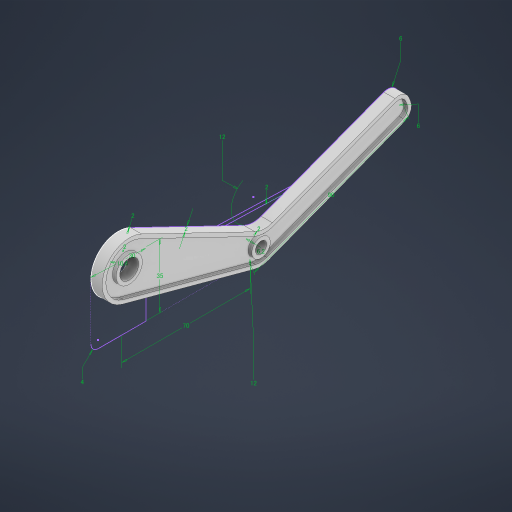
# Autodesk Inventor part: myPartbasic
Saved by Autodesk Inventor 2024.3 (Build 283343000, 343)
## iProperties
Created: 2024-11-22
Part Number: myPartbasic
Material: 一般
Document SubType Name: Modeling
Designer: ktamu
Density: 1 g/cm^3
Appearance: 既定
Author: ktamu
Autodesk Inventor part; units mm, degrees
ref_plane "YZ Plane" through (0, 0, 0) normal (1, 0, 0) x (0, 1, 0)
ref_plane "XZ Plane" through (0, 0, 0) normal (0, 1, 0) x (-1, 0, 0)
ref_plane "XY Plane" through (0, 0, 0) normal (0, 0, 1) x (1, 0, 0)
sketch "スケッチ1" plane through (0, 0, 0) normal (1, 0, 0) x (0, 1, 0)
  circle A0 centre (0, 0) radius 5.2
  circle A1 centre (0, 0) radius 7.2
  circle A2 centre (0, 0) radius 15
  line L0 (0, 15) -> (0, -15)
  line L1 (0, -15) -> (-35, -15)
  line L2 (-35, -15) -> (-35, 11)
  line L3 (-31, 15) -> (0, 15) construction
  line L4 (-35, -2) -> (-35, -69.7896) construction
  line L5 (-16.4564, -68.522) -> (13.5054, -6.5271)
  line L6 (-34.7855, -71.5009) -> (-3.0714, -155.7281) construction
  line L7 (-16.8824, -77.9722) -> (8.3603, -145.0124)
  line L8 (4.8594, -152.7418) -> (2.5202, -153.6226)
  arc A3 (-16.4564, -68.522) -> (-16.8824, -77.9722) centre (-5.6521, -73.7437) ccw
  line L9 (-11.5149, -58.2973) -> (-12.5354, -89.5169)
  line L10 (-9.3687, -53.8565) -> (-10.6942, -94.4069)
  arc A4 (-31, 15) -> (-35, 11) centre (-31, 11) ccw
  line L11 (-33.9826, -68.2361) -> (-14.4803, 3.9141)
  line L12 (-33.6108, -75.6431) -> (-5.2003, -150.1454)
  arc A5 (-33.9826, -68.2361) -> (-33.6108, -75.6431) centre (-22.3983, -71.3674) ccw
  circle A6 centre (-25.7133, -72) radius 3.1
  circle A7 centre (-25.7133, -72) radius 5.1
  circle A8 centre (0, 0) radius 13
  arc A9 (4.8594, -152.7418) -> (8.3603, -145.0124) centre (2.7452, -147.1267) ccw
  arc A10 (-5.2003, -150.1454) -> (2.5202, -153.6226) centre (0.4059, -148.0075) ccw
  line L13 (11.7047, -5.6568) -> (-18.2572, -67.6517)
  arc A11 (-18.2572, -67.6517) -> (-18.7541, -78.677) centre (-5.6521, -73.7437) ccw
  line L14 (-18.7541, -78.677) -> (6.4886, -145.7172)
  arc A12 (4.1547, -150.8701) -> (6.4886, -145.7172) centre (2.7452, -147.1267) ccw
  line L15 (4.1547, -150.8701) -> (1.8154, -151.7509)
  arc A13 (-3.3316, -149.4327) -> (1.8154, -151.7509) centre (0.4059, -148.0075) ccw
  line L16 (-3.3316, -149.4327) -> (-31.742, -74.9304)
  arc A14 (-32.0519, -68.758) -> (-31.742, -74.9304) centre (-22.3983, -71.3674) ccw
  line L17 (-32.0519, -68.758) -> (-12.5496, 3.3922)
  point P0 (-35, -72)
  point P1 (-12.5496, 3.3922)
  dimension "d0" = 10.4
  dimension "d1" = 2
  dimension "d2" = 30
  dimension "d3" = 35
  dimension "d4" = 70
  dimension "d6" = 90
  dimension "d8" = 12
  dimension "d9" = 2
  dimension "d10" = 4
  dimension "d11" = 12
  dimension "d12" = 6.2
  dimension "d13" = 2
  dimension "d14" = 2
  dimension "d15" = 6
  dimension "d16" = 6
  dimension "d17" = 2
  constraints: 36 end point, 22 point on circle, 15 centre point, 12 tangent, 9 point on line, 5 coincident, 4 parallel, 3 perpendicular, 2 vertical, 1 midpoint, 8 other
  measures "d0" diameter of A0
  measures "d1" radial gap between concentric circles of A1 A0
  measures "d2" diameter of A2
  measures "d3" distance of L0.end L1.end
  measures "d4" distance of L4.start point (-35, -72)
  measures "d6" distance of L6.start L6.end
  measures "d8" radius of A3
  measures "d9" distance between parallel lines of L10 L9
  measures "d10" radius of A4
  measures "d11" radius of A5
  measures "d12" diameter of A6
  measures "d13" radial gap between concentric circles of A7 A6
  measures "d14" radial gap between concentric circles of A2 A8
  measures "d15" radius of A9
  measures "d16" radius of A10
  measures "d17" distance between parallel lines of L5 L13
extrude "押し出し1" add sketch "スケッチ1" along normal blind 6.2 contours A8 L17 A2 L0 | L0 A2 L13 A8 | A2 L17 L1 L11 | A2 L5 A3 L7 A9 L8 A10 L12 A5 L11 L1 L17 A14 L16 A13 L15 A12 L14 A11 L13 picked at (-13.9996, -0.5672) picked at (10.2069, -9.5984)
extrude "押し出し2" add sketch "スケッチ1" along normal blind 6 contours A0 L0 A1 | A0 L0 A1
extrude "押し出し3" add sketch "スケッチ1" along normal blind 4 contours L0 A8 A1 | A1 L0 A8 | A8 L13 A2 L0 | L0 A2 L17 A8 | L1 L17 A2 | A2 L13 A11 L14 A12 L15 A13 L16 A14 L17 L1 picked at (7.3931, -11.427) picked at (-1.085, -14.2142)
extrude "押し出し4" add sketch "スケッチ1" along normal blind 6 contours A7
